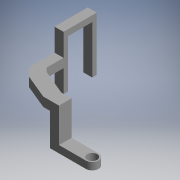
# Autodesk Inventor part: armv3
Saved by Autodesk Inventor 2019 (Build 230136000, 136)
## iProperties
Created: 2020-04-01
Part Number: armv3
Material: Generic
Document SubType Name: Modeling
Designer: Pulag
Density: 1 g/cm^3
Appearance: Default
Author: Pulag
Autodesk Inventor part; units mm, degrees
ref_plane "YZ Plane" through (0, 0, 0) normal (1, 0, 0) x (0, 1, 0)
ref_plane "XZ Plane" through (0, 0, 0) normal (0, 1, 0) x (-1, 0, 0)
ref_plane "Work Plane7" through (19.7548, -26.2861, 10.5259) normal (0, -1, 0) x (1, 0, 0)
sketch "Sketch10" plane through (0, 0, 0) normal (0, 1, 0) x (-1, 0, 0)
  line L0 (-27.0112, 18.5709) -> (-26.4391, 18.8263) projected
  line L1 (-25.8204, 18.925) -> (-26.4391, 18.8263) projected
  line L2 (-25.1972, 18.8603) -> (-25.8204, 18.925) projected
  line L3 (-24.6121, 18.6364) -> (-25.1972, 18.8603) projected
  line L4 (-24.1048, 18.2687) -> (-24.6121, 18.6364) projected
  line L5 (-23.7099, 17.7823) -> (-24.1048, 18.2687) projected
  line L6 (-23.4545, 17.2102) -> (-23.7099, 17.7823) projected
  line L7 (-23.4545, 17.2102) -> (-23.3557, 16.5915) projected
  line L8 (-23.4205, 15.9683) -> (-23.3557, 16.5915) projected
  line L9 (-23.4205, 15.9683) -> (-23.6444, 15.3832) projected
  line L10 (-23.6444, 15.3832) -> (-24.0121, 14.8759) projected
  line L11 (-24.0121, 14.8759) -> (-24.4985, 14.481) projected
  line L12 (-24.4985, 14.481) -> (-25.0706, 14.2256) projected
  line L13 (-25.0706, 14.2256) -> (-25.6893, 14.1268) projected
  line L14 (-25.6893, 14.1268) -> (-26.3125, 14.1916) projected
  line L15 (-26.3125, 14.1916) -> (-26.8976, 14.4155) projected
  line L16 (-26.8976, 14.4155) -> (-27.4049, 14.7832) projected
  line L17 (-27.4049, 14.7832) -> (-27.7998, 15.2696) projected
  line L18 (-28.0552, 15.8417) -> (-27.7998, 15.2696) projected
  line L19 (-28.0552, 15.8417) -> (-28.1539, 16.4604) projected
  line L20 (-28.1539, 16.4604) -> (-28.0892, 17.0836) projected
  line L21 (-28.0892, 17.0836) -> (-27.8653, 17.6687) projected
  line L22 (-27.8653, 17.6687) -> (-27.4976, 18.176) projected
  line L23 (-27.0112, 18.5709) -> (-27.4976, 18.176) projected
  line L24 (-26.7545, 16.4986) -> (-26.7275, 16.7583) projected
  line L25 (-26.7133, 16.2408) -> (-26.7545, 16.4986) projected
  line L26 (-26.6069, 16.0025) -> (-26.7133, 16.2408) projected
  line L27 (-26.4424, 15.7998) -> (-26.6069, 16.0025) projected
  line L28 (-26.231, 15.6466) -> (-26.4424, 15.7998) projected
  line L29 (-25.9872, 15.5533) -> (-26.231, 15.6466) projected
  line L30 (-25.7275, 15.5263) -> (-25.9872, 15.5533) projected
  line L31 (-25.4697, 15.5675) -> (-25.7275, 15.5263) projected
  line L32 (-25.2314, 15.6739) -> (-25.4697, 15.5675) projected
  line L33 (-25.0287, 15.8384) -> (-25.2314, 15.6739) projected
  line L34 (-24.8755, 16.0498) -> (-25.0287, 15.8384) projected
  line L35 (-24.7822, 16.2936) -> (-24.8755, 16.0498) projected
  line L36 (-24.7552, 16.5533) -> (-24.7822, 16.2936) projected
  line L37 (-24.7552, 16.5533) -> (-24.7963, 16.8111) projected
  line L38 (-24.7963, 16.8111) -> (-24.9028, 17.0494) projected
  line L39 (-24.9028, 17.0494) -> (-25.0673, 17.2521) projected
  line L40 (-25.0673, 17.2521) -> (-25.2787, 17.4053) projected
  line L41 (-25.2787, 17.4053) -> (-25.5225, 17.4986) projected
  line L42 (-25.5225, 17.4986) -> (-25.7822, 17.5256) projected
  line L43 (-25.7822, 17.5256) -> (-26.04, 17.4844) projected
  line L44 (-26.04, 17.4844) -> (-26.2783, 17.378) projected
  line L45 (-26.2783, 17.378) -> (-26.481, 17.2135) projected
  line L46 (-26.481, 17.2135) -> (-26.6342, 17.0021) projected
  line L47 (-26.6342, 17.0021) -> (-26.7275, 16.7583) projected
  line L48 (-27.0112, 18.5709) -> (-26.4391, 18.8263) projected
  line L49 (-25.8204, 18.925) -> (-26.4391, 18.8263) projected
  line L50 (-25.1972, 18.8603) -> (-25.8204, 18.925) projected
  line L51 (-24.6121, 18.6364) -> (-25.1972, 18.8603) projected
  line L52 (-24.1048, 18.2687) -> (-24.6121, 18.6364) projected
  line L53 (-23.7099, 17.7823) -> (-24.1048, 18.2687) projected
  line L54 (-23.4545, 17.2102) -> (-23.7099, 17.7823) projected
  line L55 (-23.4545, 17.2102) -> (-23.3557, 16.5915) projected
  line L56 (-23.4205, 15.9683) -> (-23.3557, 16.5915) projected
  line L57 (-23.4205, 15.9683) -> (-23.6444, 15.3832) projected
  line L58 (-23.6444, 15.3832) -> (-24.0121, 14.8759) projected
  line L59 (-24.0121, 14.8759) -> (-24.4985, 14.481) projected
  line L60 (-24.4985, 14.481) -> (-25.0706, 14.2256) projected
  line L61 (-25.0706, 14.2256) -> (-25.6893, 14.1268) projected
  line L62 (-25.6893, 14.1268) -> (-26.3125, 14.1916) projected
  line L63 (-26.3125, 14.1916) -> (-26.8976, 14.4155) projected
  line L64 (-26.8976, 14.4155) -> (-27.4049, 14.7832) projected
  line L65 (-27.4049, 14.7832) -> (-27.7998, 15.2696) projected
  line L66 (-28.0552, 15.8417) -> (-27.7998, 15.2696) projected
  line L67 (-28.0552, 15.8417) -> (-28.1539, 16.4604) projected
  line L68 (-28.1539, 16.4604) -> (-28.0892, 17.0836) projected
  line L69 (-28.0892, 17.0836) -> (-27.8653, 17.6687) projected
  line L70 (-27.8653, 17.6687) -> (-27.4976, 18.176) projected
  line L71 (-27.0112, 18.5709) -> (-27.4976, 18.176) projected
  line L72 (-26.7545, 16.4986) -> (-26.7275, 16.7583) projected
  line L73 (-26.7133, 16.2408) -> (-26.7545, 16.4986) projected
  line L74 (-26.6069, 16.0025) -> (-26.7133, 16.2408) projected
  line L75 (-26.4424, 15.7998) -> (-26.6069, 16.0025) projected
  line L76 (-26.231, 15.6466) -> (-26.4424, 15.7998) projected
  line L77 (-25.9872, 15.5533) -> (-26.231, 15.6466) projected
  line L78 (-25.7275, 15.5263) -> (-25.9872, 15.5533) projected
  line L79 (-25.4697, 15.5675) -> (-25.7275, 15.5263) projected
  line L80 (-25.2314, 15.6739) -> (-25.4697, 15.5675) projected
  line L81 (-25.0287, 15.8384) -> (-25.2314, 15.6739) projected
  line L82 (-24.8755, 16.0498) -> (-25.0287, 15.8384) projected
  line L83 (-24.7822, 16.2936) -> (-24.8755, 16.0498) projected
  line L84 (-24.7552, 16.5533) -> (-24.7822, 16.2936) projected
  line L85 (-24.7552, 16.5533) -> (-24.7963, 16.8111) projected
  line L86 (-24.7963, 16.8111) -> (-24.9028, 17.0494) projected
  line L87 (-24.9028, 17.0494) -> (-25.0673, 17.2521) projected
  line L88 (-25.0673, 17.2521) -> (-25.2787, 17.4053) projected
  line L89 (-25.2787, 17.4053) -> (-25.5225, 17.4986) projected
  line L90 (-25.5225, 17.4986) -> (-25.7822, 17.5256) projected
  line L91 (-25.7822, 17.5256) -> (-26.04, 17.4844) projected
  line L92 (-26.04, 17.4844) -> (-26.2783, 17.378) projected
  line L93 (-26.2783, 17.378) -> (-26.481, 17.2135) projected
  line L94 (-26.481, 17.2135) -> (-26.6342, 17.0021) projected
  line L95 (-26.6342, 17.0021) -> (-26.7275, 16.7583) projected
  circle A0 centre (-25.7548, 16.5259) radius 2.75
  arc A1 (-25.7548, 20.0259) -> (-25.7548, 13.0259) centre (-25.7548, 16.5259) ccw
  line L96 (-25.7548, 20.0259) -> (-5.7548, 20.0259) construction
  line L97 (-25.7548, 13.0259) -> (-5.7548, 13.0259)
  line L98 (-5.7548, 13.0259) -> (-5.7548, 20.0259)
  line L99 (-25.7548, 20.0259) -> (-5.7548, 20.0259)
  point P0 (0, 0)
  dimension "d36" = 5.5
  dimension "d37" = 7
  dimension "d40" = 20
  constraints: 8 end point, 3 horizontal, 2 centre point, 2 point on circle, 1 coincident, 1 perpendicular
  measures "d36" diameter of A0
  measures "d37" diameter of A1
  measures "d40" distance of L97.start L97.end
extrude "Extrusion8" add sketch "Sketch10" against normal blind 4 from surface at -26.2861 contours L99 L98 L97 A1
sketch "Sketch12" plane through (0, 0, 0) normal (0, 1, 0) x (-1, 0, 0)
  line L0 (26.2, -19.75) -> (26.2, -7.25) projected
  line L1 (26.2, -19.75) -> (11, -19.75) projected
  line L2 (11, -7.25) -> (11, -19.75) projected
  line L3 (11, -7.25) -> (26.2, -7.25) projected
  line L4 (22.4706, -11.917) -> (22.6, -11.9) projected
  line L5 (22.35, -11.967) -> (22.4706, -11.917) projected
  line L6 (22.2464, -12.0464) -> (22.35, -11.967) projected
  line L7 (22.167, -12.15) -> (22.2464, -12.0464) projected
  line L8 (22.117, -12.2706) -> (22.167, -12.15) projected
  line L9 (22.1, -12.4) -> (22.117, -12.2706) projected
  line L10 (22.117, -12.5294) -> (22.1, -12.4) projected
  line L11 (22.167, -12.65) -> (22.117, -12.5294) projected
  line L12 (22.2464, -12.7536) -> (22.167, -12.65) projected
  line L13 (22.35, -12.833) -> (22.2464, -12.7536) projected
  line L14 (22.35, -12.833) -> (22.4706, -12.883) projected
  line L15 (22.4706, -12.883) -> (22.6, -12.9) projected
  line L16 (22.6, -12.9) -> (22.7294, -12.883) projected
  line L17 (22.85, -12.833) -> (22.7294, -12.883) projected
  line L18 (22.9536, -12.7536) -> (22.85, -12.833) projected
  line L19 (23.033, -12.65) -> (22.9536, -12.7536) projected
  line L20 (23.033, -12.65) -> (23.083, -12.5294) projected
  line L21 (23.083, -12.5294) -> (23.1, -12.4) projected
  line L22 (23.1, -12.4) -> (23.083, -12.2706) projected
  line L23 (23.083, -12.2706) -> (23.033, -12.15) projected
  line L24 (23.033, -12.15) -> (22.9536, -12.0464) projected
  line L25 (22.9536, -12.0464) -> (22.85, -11.967) projected
  line L26 (22.85, -11.967) -> (22.7294, -11.917) projected
  line L27 (22.6, -11.9) -> (22.7294, -11.917) projected
  line L28 (22.4706, -13.017) -> (22.6, -13) projected
  line L29 (22.35, -13.067) -> (22.4706, -13.017) projected
  line L30 (22.2464, -13.1464) -> (22.35, -13.067) projected
  line L31 (22.167, -13.25) -> (22.2464, -13.1464) projected
  line L32 (22.117, -13.3706) -> (22.167, -13.25) projected
  line L33 (22.1, -13.5) -> (22.117, -13.3706) projected
  line L34 (22.117, -13.6294) -> (22.1, -13.5) projected
  line L35 (22.167, -13.75) -> (22.117, -13.6294) projected
  line L36 (22.2464, -13.8536) -> (22.167, -13.75) projected
  line L37 (22.35, -13.933) -> (22.2464, -13.8536) projected
  line L38 (22.35, -13.933) -> (22.4706, -13.983) projected
  line L39 (22.4706, -13.983) -> (22.6, -14) projected
  line L40 (22.6, -14) -> (22.7294, -13.983) projected
  line L41 (22.85, -13.933) -> (22.7294, -13.983) projected
  line L42 (22.9536, -13.8536) -> (22.85, -13.933) projected
  line L43 (23.033, -13.75) -> (22.9536, -13.8536) projected
  line L44 (23.033, -13.75) -> (23.083, -13.6294) projected
  line L45 (23.083, -13.6294) -> (23.1, -13.5) projected
  line L46 (23.1, -13.5) -> (23.083, -13.3706) projected
  line L47 (23.083, -13.3706) -> (23.033, -13.25) projected
  line L48 (23.033, -13.25) -> (22.9536, -13.1464) projected
  line L49 (22.9536, -13.1464) -> (22.85, -13.067) projected
  line L50 (22.85, -13.067) -> (22.7294, -13.017) projected
  line L51 (22.6, -13) -> (22.7294, -13.017) projected
  line L52 (22.4706, -14.117) -> (22.6, -14.1) projected
  line L53 (22.35, -14.167) -> (22.4706, -14.117) projected
  line L54 (22.2464, -14.2464) -> (22.35, -14.167) projected
  line L55 (22.167, -14.35) -> (22.2464, -14.2464) projected
  line L56 (22.117, -14.4706) -> (22.167, -14.35) projected
  line L57 (22.1, -14.6) -> (22.117, -14.4706) projected
  line L58 (22.117, -14.7294) -> (22.1, -14.6) projected
  line L59 (22.167, -14.85) -> (22.117, -14.7294) projected
  line L60 (22.2464, -14.9536) -> (22.167, -14.85) projected
  line L61 (22.35, -15.033) -> (22.2464, -14.9536) projected
  line L62 (22.35, -15.033) -> (22.4706, -15.083) projected
  line L63 (22.4706, -15.083) -> (22.6, -15.1) projected
  line L64 (22.6, -15.1) -> (22.7294, -15.083) projected
  line L65 (22.85, -15.033) -> (22.7294, -15.083) projected
  line L66 (22.9536, -14.9536) -> (22.85, -15.033) projected
  line L67 (23.033, -14.85) -> (22.9536, -14.9536) projected
  line L68 (23.033, -14.85) -> (23.083, -14.7294) projected
  line L69 (23.083, -14.7294) -> (23.1, -14.6) projected
  line L70 (23.1, -14.6) -> (23.083, -14.4706) projected
  line L71 (23.083, -14.4706) -> (23.033, -14.35) projected
  line L72 (23.033, -14.35) -> (22.9536, -14.2464) projected
  line L73 (22.9536, -14.2464) -> (22.85, -14.167) projected
  line L74 (22.85, -14.167) -> (22.7294, -14.117) projected
  line L75 (22.6, -14.1) -> (22.7294, -14.117) projected
  line L76 (8.5, -12.9) -> (11, -12.9) projected
  line L77 (8.5, -7.25) -> (8.5, -12.9) projected
  line L78 (8.5, -7.25) -> (11, -7.25) projected
  line L79 (11, -12.9) -> (11, -7.25) projected
  line L80 (8.5, -19.75) -> (11, -19.75) projected
  line L81 (8.5, -14.1) -> (8.5, -19.75) projected
  line L82 (8.5, -14.1) -> (11, -14.1) projected
  line L83 (11, -19.75) -> (11, -14.1) projected
  line L84 (11, -7.25) -> (16, -7.25)
  line L85 (16, -7.25) -> (16, -19.75)
  line L86 (16, -19.75) -> (11, -19.75)
  line L87 (11, -19.75) -> (11, -7.25)
  line L88 (16, -7.25) -> (11, -7.25)
  line L89 (11, -7.25) -> (11, -4.25)
  line L90 (11, -4.25) -> (16, -4.25)
  line L91 (16, -4.25) -> (16, -7.25)
  line L92 (16, -19.75) -> (11, -19.75)
  line L93 (11, -19.75) -> (11, -22.75)
  line L94 (11, -22.75) -> (16, -22.75)
  line L95 (16, -22.75) -> (16, -19.75)
  point P0 (0, 0)
  dimension "d41" = 5
  dimension "d42" = 3
  dimension "d43" = 3
  constraints: 24 end point, 6 parallel, 3 horizontal, 3 perpendicular, 3 point on line
  measures "d41" distance of L85.end L86.end
  measures "d42" distance of L88.end L89.end
  measures "d43" distance of L93.end L92.end
extrude "Extrusion10" add sketch "Sketch12" against normal blind 24.75 contours L95 L94 L93 L1 | L1 L2 L3 L85 | L3 L89 L90 L91
sketch "Sketch13" plane through (0, 0, 0) normal (0, 1, 0) x (1, 0, 0)
  line L0 (-16, 22.75) -> (-16, 4.25) projected
  line L1 (-16, 4.25) -> (-11, 4.25) projected
  line L2 (-11, 4.25) -> (-11, 22.75) projected
  line L3 (-11, 22.75) -> (-16, 22.75) projected
  point P0 (0, 0)
extrude "Extrusion11" add sketch "Sketch13" along normal blind 5.25
sketch "Sketch14" plane through (-16, -24.75, -4.25) normal (0, 0, 1) x (1, 0, 0)
  line L0 (0, 0) -> (0, 30) projected
  line L1 (5, 0) -> (0, 0) projected
  line L2 (5, 0) -> (5, 30) projected
  line L3 (0, 30) -> (5, 30) projected
  line L4 (21.7548, -5.5361) -> (41.7548, -5.5361) projected
  line L5 (41.7548, -1.5361) -> (41.7548, -5.5361) projected
  line L6 (21.7548, -1.5361) -> (41.7548, -1.5361) projected
  line L7 (21.7548, -5.5361) -> (21.7548, -1.5361) projected
  line L8 (21.7548, -5.5361) -> (26.7548, -5.5361)
  line L9 (26.7548, -5.5361) -> (26.7548, 12.4639)
  line L10 (26.7548, 12.4639) -> (21.7548, 12.4639)
  line L11 (21.7548, 12.4639) -> (21.7548, -5.5361)
  line L12 (0, 0) -> (0, 30) projected
  line L13 (26.7548, 12.4639) -> (0, 12.4639)
  line L14 (0, 12.4639) -> (0, 17.4639)
  line L15 (0, 17.4639) -> (26.7548, 17.4639)
  line L16 (26.7548, 17.4639) -> (26.7548, 12.4639)
  point P0 (16, 24.75)
  dimension "d48" = 5
  dimension "d49" = 18
  dimension "d50" = 5
  constraints: 16 end point, 4 parallel, 2 horizontal, 2 perpendicular, 1 point on line
  measures "d48" distance of L10.end L9.end
  measures "d49" distance of L9.end L8.end
  measures "d50" distance of L13.end L14.end
extrude "Extrusion12" add sketch "Sketch14" along normal up to surface (7 mm away) from surface at 17.2759 contours L0 L15 L2 L13 | L2 L15 L16 L10 L13 | L10 L9 L6 L11 | L6 L9 L4 L7
sketch "Sketch15" plane through (-16, -24.75, -4.25) normal (0, 0, 1) x (1, 0, 0)
  line L0 (41.7548, -1.5361) -> (26.7548, -1.5361) projected
  line L1 (41.7548, -5.5361) -> (41.7548, -1.5361) projected
  line L2 (41.7548, -5.5361) -> (21.7548, -5.5361) projected
  line L3 (21.7548, 12.4639) -> (21.7548, -5.5361) projected
  line L4 (0, 12.4639) -> (21.7548, 12.4639) projected
  line L5 (0, 17.4639) -> (0, 12.4639) projected
  line L6 (26.7548, 17.4639) -> (0, 17.4639) projected
  line L7 (26.7548, -1.5361) -> (26.7548, 17.4639) projected
  line L8 (0, 0) -> (0, 30) projected
  line L9 (5, 0) -> (0, 0) projected
  line L10 (5, 0) -> (5, 30) projected
  line L11 (0, 30) -> (5, 30) projected
  line L12 (0, 17.4639) -> (5, 17.4639)
  line L13 (5, 17.4639) -> (5, 12.4639)
  line L14 (5, 12.4639) -> (0, 12.4639)
  line L15 (0, 12.4639) -> (0, 17.4639)
  point P0 (16, 24.75)
  point P1 (2.919, 35.6962)
  constraints: 8 end point, 2 parallel, 2 point on line, 1 horizontal, 1 perpendicular, 1 other
extrude "Extrusion13" add sketch "Sketch15" along normal up to surface (17.2759 mm away) contours L10 L4 L5 L6
sketch "Sketch16" plane through (-16, -24.75, -22.75) normal (-1, 0, 0) x (0, 0, 1)
  line L0 (3, 3.4417) -> (15.5, 3.4417) projected
  line L1 (15.5, 3.4417) -> (15.5, 25.9417) projected
  line L2 (15.5, 25.9417) -> (3, 25.9417) projected
  line L3 (3, 3.4417) -> (3, 25.9417) projected
  line L4 (3, 25.9417) -> (15.5, 3.4417)
  line L5 (2.5, 2.6917) -> (16, 2.6917)
  line L6 (16, 2.6917) -> (16, 26.6917)
  line L7 (16, 26.6917) -> (2.5, 26.6917)
  line L8 (2.5, 26.6917) -> (2.5, 2.6917)
  line L9 (2.5, 2.6917) -> (16, 26.6917) construction
  line L10 (16, 2.6917) -> (2.5, 26.6917) construction
  line L11 (2.5, 2.6917) -> (16, 2.6917)
  line L12 (16, 2.6917) -> (16, -0.068)
  line L13 (16, -0.068) -> (2.5, -0.068)
  line L14 (2.5, -0.068) -> (2.5, 2.6917)
  point P0 (22.75, 24.75)
  point P1 (9.25, 14.6917)
  dimension "d55" = 13.5
  dimension "d56" = 24
  constraints: 22 end point, 4 parallel, 3 midpoint, 2 horizontal, 2 perpendicular
  measures "d55" distance of L7.end L6.end
  measures "d56" distance of L6.end L5.end
extrude "Extrusion14" cut sketch "Sketch16" against normal up to surface (5 mm away) contours L3 L4 L0 | L4 L2 L1 | L8 L7 L6 L5 | L5 L12 L13 L14
chamfer "Chamfer1" distance 10 angle 45 1 edges at (-16, -9.7861, 20.0259)
chamfer "Chamfer2" distance 8 angle 45 1 edges at (-11, -9.7861, 13.0259)
chamfer "Chamfer3" distance 8 angle 45 1 edges at (-6, -9.7861, 20.0259)
chamfer "Chamfer4" distance 8 angle 45 1 edges at (-3, -9.7861, 13.0259)
body "Solid2"
